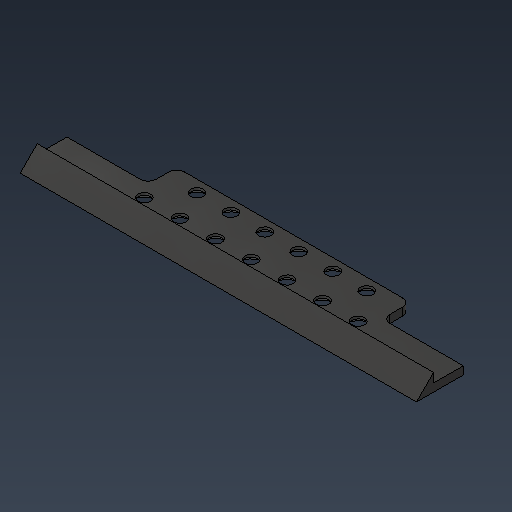
# Autodesk Inventor part: Plog2
Saved by Autodesk Inventor 2026.2 (Build 302298010, 298A)
## iProperties
Created: 2022-01-27
Part Number: Plog2
Material: Steel, Carbon
Document SubType Name: Modeling
Designer: Michał
Density: 7.85 g/cm^3
Appearance: Dark Gray
Mass: 23.2729 g
Surface Area: 39.2273 cm^2
Volume: 2.9647 cm^3
Author: Michał
Autodesk Inventor part; units mm, degrees
ref_plane "YZ Plane" through (0, 0, 0) normal (1, 0, 0) x (0, 1, 0)
ref_plane "XZ Plane" through (0, 0, 0) normal (0, 1, 0) x (-1, 0, 0)
ref_plane "XY Plane" through (0, 0, 0) normal (0, 0, 1) x (1, 0, 0)
sketch "Szkic1" plane through (0, 0, 0) normal (1, 0, 0) x (0, 1, 0)
  line L0 (0, 0) -> (2, -2)
  line L1 (2, -2) -> (2, -19)
  line L2 (2, -19) -> (0, -19)
  line L3 (0, -19) -> (0, -2)
  line L4 (0, -2) -> (0, 0)
  line L5 (0, -2) -> (2, -2)
  line L6 (2, -2) -> (4.3, -4.3)
  line L7 (4.3, -4.3) -> (2, -4.3)
  line L8 (2, -2) -> (4.3, -4.3)
  line L9 (4.3, -4.3) -> (2, -4.3)
  line L10 (4, -4) -> (4, -4.3) construction
  line L11 (4, -4) -> (2, -4) construction
  point P0 (5, -5)
  dimension "d1" = 2
  dimension "d2" = 45
  dimension "d44" = 45
  dimension "d45" = 2
  dimension "d46" = 17
  dimension "d50" = -4.3
  dimension "d51" = 19
  dimension "d54" = 0
  dimension "d98" = 2.3
  dimension "d125" = 4
  dimension "d126" = 0.3
  constraints: 24 end point, 9 point on line, 7 perpendicular, 1 coincident, 1 horizontal, 1 vertical, 2 other
  measures "d1" distance between parallel lines of L4 L1
  measures "d2" angle of L4 L0
  measures "d44" angle of L7 L6
  measures "d45" distance of L3.end L0.start
  measures "d46" distance of L2.end L3.end
  measures "d51" distance from line of L2 L0.start
  measures "d98" distance from line of L1 L6.end
  measures "d125" distance between parallel lines of L3 L10
  measures "d126" distance between parallel lines of L7 L11
extrude "Wyciągnięcie proste1" add sketch "Szkic1" along normal mid plane 100
sketch "Sketch4" plane through (-50, 0, -19) normal (0, -1, 0) x (1, 0, 0)
  line L0 (0, 0) -> (0, 19) projected
  line L1 (0, 0) -> (100, 0) projected
  line L2 (100, 19) -> (100, 0) projected
  line L3 (100, 19) -> (0, 19) projected
  line L4 (80, 0) -> (80, 19)
  line L5 (100, 19) -> (50, 19) projected
  line L6 (20, 19) -> (20, 0)
  line L7 (0, 0) -> (100, 0) projected
  line L8 (0, 14.7) -> (100, 14.7) projected
  circle A0 centre (77, 10.7) radius 3
  circle A1 centre (68, 10.7) radius 3
  circle A2 centre (32, 10.7) radius 3
  circle A3 centre (23, 10.7) radius 3
  line L9 (80, 10.7) -> (20, 10.7)
  circle A4 centre (59, 10.7) radius 3.25
  circle A5 centre (71.4286, 3) radius 3
  circle A6 centre (37.1429, 3) radius 3
  circle A7 centre (28.5714, 3) radius 3
  line L10 (80, 3) -> (20, 3)
  circle A8 centre (62.8571, 3) radius 3
  circle A9 centre (41, 10.7) radius 3
  circle A10 centre (50, 10.7) radius 3
  circle A11 centre (45.7143, 3) radius 3
  circle A12 centre (54.2857, 3) radius 3
  dimension "d67" = 6
  dimension "d70" = 6
  dimension "d22" = 20
  dimension "d23" = 20
  dimension "d68" = 6
  dimension "d69" = 6
  dimension "d72" = 9
  dimension "d75" = 9
  dimension "d104" = 6.5
  dimension "d106" = 9
  dimension "d109" = 6
  dimension "d110" = 6
  dimension "d111" = 6
  dimension "d113" = 8.5714
  dimension "d114" = 6
  dimension "d115" = 8.5714
  dimension "d119" = 1
  dimension "d122" = 8.5714
  dimension "d123" = 8.5714
  dimension "d124" = 3
  dimension "d127" = 6
  dimension "d128" = 6
  dimension "d129" = 9
  dimension "d130" = 9
  dimension "d131" = 9
  dimension "d132" = 6
  dimension "d133" = 6
  dimension "d134" = 8.5714
  dimension "d135" = 8.5714
  dimension "d136" = 8.5714
  constraints: 11 centre point, 11 point on line, 6 end point, 2 horizontal alignment, 2 perpendicular, 2 vertical, 1 horizontal, 14 other
  measures "d22" distance between parallel lines of L2 L4
  measures "d23" distance between parallel lines of L0 L6
  measures "d68" diameter of A1
  measures "d69" diameter of A2
  measures "d72" distance of A1.centre point (77, 10.7)
  measures "d75" distance of point (23, 10.7) A2.centre
  measures "d104" diameter of A4
  measures "d106" distance of A1.centre A4.centre
  measures "d109" diameter of A5
  measures "d110" diameter of A6
  measures "d111" diameter of A7
  measures "d113" distance of A7.centre A6.centre
  measures "d114" diameter of A8
  measures "d115" distance of A5.centre A8.centre
  measures "d122" distance from line of A5.centre L4
  measures "d123" distance from line of L6 A7.centre
  measures "d124" distance from line of A5.centre L1
  measures "d127" diameter of A9
  measures "d128" diameter of A10
  measures "d129" distance of A9.centre A2.centre
  measures "d130" distance of A10.centre A9.centre
  measures "d131" distance of A10.centre A4.centre
  measures "d132" diameter of A11
  measures "d133" diameter of A12
  measures "d134" distance of A12.centre A8.centre
  measures "d135" distance of A12.centre A11.centre
  measures "d136" distance of A11.centre A6.centre
hole "Hole2" at (27, 0, -8.3) at (18, 0, -8.3) at (-18, 0, -8.3) at (-27, 0, -8.3) at (9, 0, -8.3) at (-21.4286, 0, -16) at (-12.8571, 0, -16) at (12.8571, 0, -16) at (21.4286, 0, -16) at (-9, 0, -8.3) at (-4.2857, 0, -16) at (0, 0, -8.3) at (4.2857, 0, -16) direction (0, 1, 0) diameter 3.2 depth 8.8 countersink diameter 6 countersink angle 90 clearance for "Countersunk Flat Head Screw ISO 2009/7046" size "M3" standard "ISO"
sketch "Sketch5" plane through (-50, 0, 0) normal (0, -1, 0) x (1, 0, 0)
  line L0 (100, 0) -> (100, -19) projected
  line L1 (100, 0) -> (0, 0) projected
  line L2 (0, -19) -> (0, 0) projected
  line L3 (100, -11.808) -> (79.5, -11.808)
  line L4 (79.5, -11.808) -> (79.5, -28.94)
  line L5 (79.5, -28.94) -> (100, -28.94)
  line L6 (100, -28.94) -> (100, -11.808)
  line L7 (0, -19) -> (20.5, -19)
  line L8 (20.5, -19) -> (20.5, -11.808)
  line L9 (20.5, -11.808) -> (0, -11.808)
  line L10 (0, -11.808) -> (0, -19)
  circle A0 centre (23, -8.3) radius 3 projected
  circle A1 centre (32, -8.3) radius 3 projected
  circle A2 centre (68, -8.3) radius 3 projected
  circle A3 centre (77, -8.3) radius 3 projected
  circle A4 centre (59, -8.3) radius 3 projected
  circle A5 centre (62.8571, -16) radius 3 projected
  circle A6 centre (37.1429, -16) radius 3 projected
  circle A7 centre (71.4286, -16) radius 3 projected
  circle A8 centre (28.5714, -16) radius 3 projected
  line L11 (0, -19) -> (28.5714, -19) projected
  line L12 (28.5714, -19) -> (37.1429, -19) projected
  line L13 (37.1429, -19) -> (45.7143, -19) projected
  line L14 (62.8571, -19) -> (71.4286, -19) projected
  line L15 (71.4286, -19) -> (100, -19) projected
  circle A9 centre (45.7143, -16) radius 3 projected
  line L16 (45.7143, -19) -> (54.2857, -19) projected
  circle A10 centre (54.2857, -16) radius 3 projected
  line L17 (54.2857, -19) -> (62.8571, -19) projected
  point P0 (50, 0)
  point P1 (0, -11.808)
  point P2 (100, -30)
  dimension "d55" = 20.5
  dimension "d56" = 20.5
  dimension "d61" = 11.808
  dimension "d62" = 11.808
  constraints: 16 end point, 6 vertical alignment, 4 parallel, 2 horizontal, 2 perpendicular, 1 point on line
  measures "d55" distance of L8.end L9.end
  measures "d56" distance of L3.start L3.end
  measures "d61" distance between parallel lines of L1 L9
  measures "d62" distance between parallel lines of L1 L3
extrude "Extrusion5" cut sketch "Sketch5" against normal through all contours L0 L15 L4 L3 | L6 L5 L4 L15 | L9 L8 L7 L2
fillet "Fillet2" radius 2 4 edges at (29.5, 1, -11.808) (-29.5, 1, -11.808) (-29.5, 1, -19) (29.5, 1, -19)
equation "\"d23\" = d22"
equation "\"d72\" = d75"
equation "\"d56\" = d55"
equation "\"d62\" = d61"
equation "\"d64\" = d80"
equation "\"d79\" = d64"
equation "\"d80\" = 4.648267"
